Autodesk Inventor part; units mm, degrees
(part 4 of 4)
equation "\"d4\" = ipg"
equation "\"d5\" = ipg"
equation "\"d6\" = ipg"
equation "\"d7\" = ipg"
equation "\"d8\" = ipg"
equation "\"d9\" = ipg"
equation "\"d10\" = ipg"
equation "\"d11\" = ipg"
equation "\"d12\" = ipg"
equation "\"d13\" = ipg"
equation "\"d14\" = ipg"
equation "\"d15\" = ipg"
equation "\"d16\" = ipg"
equation "\"d17\" = ipg"
equation "\"d18\" = ipg"
equation "\"d19\" = ipg"
equation "\"d20\" = ipg"
equation "\"d21\" = ipg"
equation "\"d22\" = sw"
equation "\"d23\" = sw"
equation "\"d24\" = sw"
equation "\"d25\" = sw"
equation "\"d26\" = sw"
equation "\"d27\" = sw"
equation "\"d28\" = sw"
equation "\"d29\" = sw"
equation "\"d30\" = sw"
equation "\"d31\" = sw"
equation "\"d32\" = sw"
equation "\"d33\" = sw"
equation "\"d34\" = sw"
equation "\"d35\" = sw"
equation "\"d36\" = sw"
equation "\"d37\" = sw"
equation "\"d38\" = sw"
equation "\"d39\" = sw"
equation "\"d40\" = sw"
equation "\"d41\" = sw"
equation "\"d42\" = sw"
equation "\"d43\" = sw"
equation "\"d44\" = sw"
equation "\"d45\" = sw"
equation "\"d46\" = sw"
equation "\"d47\" = sw"
equation "\"d48\" = sw"
equation "\"d49\" = sw"
equation "\"d50\" = sw"
equation "\"d51\" = sw"
equation "\"d52\" = sw"
equation "\"d53\" = sw"
equation "\"d54\" = sw"
equation "\"d55\" = sw"
equation "\"d56\" = sw"
equation "\"d57\" = sw"
equation "\"d58\" = sw"
equation "\"d59\" = sw"
equation "\"d60\" = sw"
equation "\"d61\" = sw"
equation "\"d62\" = sw"
equation "\"d63\" = sw"
equation "\"d64\" = sw"
equation "\"sw\" = 14.005"
equation "\"ipg\" = 0.1"
body "Solid1"
